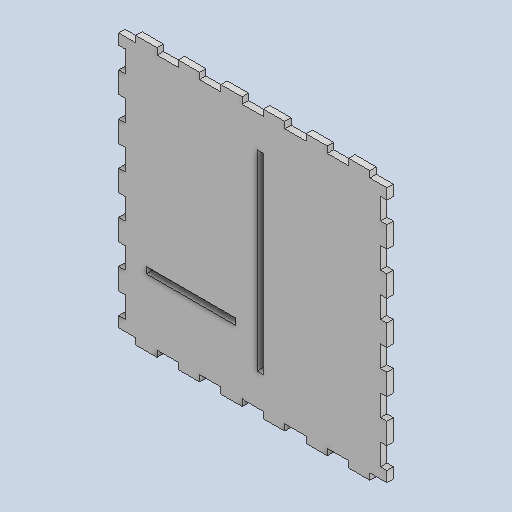
# Autodesk Inventor part: bottom
Saved by Autodesk Inventor 2022 (Build 260153000, 153)
## iProperties
Created: 2022-05-12
Part Number: bottom
Material: Generic
Document SubType Name: Modeling
Designer: Jeanette Guo
Density: 1 g/cm^3
Appearance: Default
Author: Jeanette Guo
Autodesk Inventor part; units mm, degrees
ref_plane "YZ Plane" through (0, 0, 0) normal (1, 0, 0) x (0, 1, 0)
ref_plane "XZ Plane" through (0, 0, 0) normal (0, 1, 0) x (-1, 0, 0)
ref_plane "XY Plane" through (0, 0, 0) normal (0, 0, 1) x (1, 0, 0)
sketch "Sketch2" plane through (0, 0, 0) normal (0, 0, 1) x (1, 0, 0)
  line L0 (109.6174, -113.2467) -> (109.6174, -116.2467) projected
  line L1 (106.6174, -113.2467) -> (106.6174, -116.2467) projected
  line L2 (101.6174, -113.2467) -> (109.6174, -113.2467) projected
  line L3 (101.6174, -116.2467) -> (109.6174, -116.2467) projected
  line L4 (101.6174, -113.2467) -> (101.6174, -116.2467) projected
  line L5 (106.6174, -113.2471) -> (106.6174, -108.2467) projected
  line L6 (109.6174, -113.2471) -> (109.6174, -108.2467) projected
  line L7 (106.6174, -108.2467) -> (106.6174, -98.2467) projected
  line L8 (109.6174, -108.2467) -> (109.6174, -98.2467) projected
  line L9 (109.6174, -98.2467) -> (109.6174, -88.2467) projected
  line L10 (106.6174, -98.2467) -> (106.6174, -88.2467) projected
  line L11 (106.6174, -88.2467) -> (106.6174, -78.2467) projected
  line L12 (109.6174, -88.2467) -> (109.6174, -78.2467) projected
  line L13 (109.6174, -78.2467) -> (109.6174, -68.2467) projected
  line L14 (106.6174, -78.2467) -> (106.6174, -68.2467) projected
  line L15 (106.6174, -78.2467) -> (109.6174, -78.2467) projected
  line L16 (106.6174, -88.2467) -> (109.6174, -88.2467) projected
  line L17 (106.6174, -98.2467) -> (109.6174, -98.2467) projected
  line L18 (106.6174, -108.2467) -> (109.6174, -108.2467) projected
  line L19 (91.6174, -113.2467) -> (91.6174, -116.2467) projected
  line L20 (81.6174, -113.2467) -> (81.6174, -116.2467) projected
  line L21 (71.6174, -113.2467) -> (71.6174, -116.2467) projected
  line L22 (61.6174, -113.2467) -> (61.6174, -116.2467) projected
  line L23 (51.6174, -113.2467) -> (51.6174, -116.2467) projected
  line L24 (106.6174, -68.2467) -> (109.6174, -68.2467)
  line L25 (109.6174, -108.2467) -> (106.6174, -108.2467)
  line L26 (109.6174, -98.2467) -> (106.6174, -98.2467)
  line L27 (109.6174, -88.2467) -> (106.6174, -88.2467)
  line L28 (109.6174, -78.2467) -> (106.6174, -78.2467)
  line L29 (101.6174, -113.2467) -> (101.6174, -116.2467)
  line L30 (91.6174, -113.2467) -> (91.6174, -116.2467)
  line L31 (81.6174, -113.2467) -> (81.6174, -116.2467)
  line L32 (71.6174, -113.2467) -> (71.6174, -116.2467)
  line L33 (61.6174, -113.2467) -> (61.6174, -116.2467)
  line L34 (51.6174, -113.2467) -> (51.6174, -116.2467)
  line L35 (106.6174, -113.2471) -> (106.6174, -113.2467)
  line L36 (106.6174, -113.2467) -> (106.6174, -113.2471)
  line L37 (109.6174, -108.2467) -> (109.6174, -113.2467)
  line L38 (106.6174, -98.2467) -> (106.6174, -108.2467)
  line L39 (106.6174, -108.2467) -> (106.6174, -98.2467)
  line L40 (106.6174, -88.2467) -> (106.6174, -78.2467)
  line L41 (109.6174, -68.2467) -> (109.6174, -78.2467)
  line L42 (109.6174, -88.2467) -> (109.6174, -98.2467)
  line L43 (106.6174, -78.2467) -> (106.6174, -88.2467)
  line L44 (101.6174, -113.2471) -> (106.6174, -113.2471)
  line L45 (101.6174, -116.2467) -> (91.6174, -116.2467)
  line L46 (61.6174, -113.2467) -> (71.6174, -113.2468)
  line L47 (81.6174, -113.2469) -> (91.6174, -113.247)
  line L48 (81.6174, -116.2467) -> (71.6174, -116.2467)
  line L49 (61.6174, -116.2467) -> (51.6174, -116.2467)
  line L50 (106.6174, -53.2467) -> (82.6898, -53.2467) construction
  line L51 (46.6174, -113.2467) -> (46.6174, -98.2467) construction
  line L52 (-8.3826, -113.2467) -> (-8.3826, -116.2467)
  line L53 (1.6174, -113.2467) -> (1.6174, -116.2467)
  line L54 (11.6174, -113.2467) -> (11.6174, -116.2467)
  line L55 (21.6174, -113.2467) -> (21.6174, -116.2467)
  line L56 (31.6174, -113.2467) -> (31.6174, -116.2467)
  line L57 (41.6174, -113.2467) -> (41.6174, -116.2467)
  line L58 (-8.3826, -113.2467) -> (-8.3826, -116.2467)
  line L59 (1.6174, -113.2467) -> (1.6174, -116.2467)
  line L60 (11.6174, -113.2467) -> (11.6174, -116.2467)
  line L61 (21.6174, -113.2467) -> (21.6174, -116.2467)
  line L62 (31.6174, -113.2467) -> (31.6174, -116.2467)
  line L63 (41.6174, -113.2467) -> (41.6174, -116.2467)
  line L64 (-8.3826, -116.2467) -> (1.6174, -116.2467)
  line L65 (11.6174, -116.2467) -> (21.6174, -116.2467)
  line L66 (31.6174, -116.2467) -> (41.6174, -116.2467)
  line L67 (-16.3826, -113.2471) -> (-16.3826, -108.2467)
  line L68 (-16.3826, -98.2467) -> (-16.3826, -88.2467)
  line L69 (-16.3826, -78.2467) -> (-16.3826, -68.2467)
  line L70 (-16.3826, -108.2467) -> (-16.3826, -113.2467)
  line L71 (-16.3826, -68.2467) -> (-16.3826, -78.2467)
  line L72 (-16.3826, -88.2467) -> (-16.3826, -98.2467)
  line L73 (109.6174, 6.7533) -> (109.6174, 6.7538)
  line L74 (106.6174, 6.7533) -> (106.6174, 6.7538)
  line L75 (101.6174, 6.7533) -> (109.6174, 6.7533)
  line L76 (101.6174, 6.7533) -> (101.6174, 9.7533)
  line L77 (106.6174, 6.7538) -> (106.6174, 6.7533)
  line L78 (109.6174, 6.7538) -> (109.6174, 1.7533)
  line L79 (106.6174, 1.7533) -> (106.6174, -8.2467)
  line L80 (109.6174, -8.2467) -> (109.6174, -18.2467)
  line L81 (106.6174, -18.2467) -> (106.6174, -28.2467)
  line L82 (109.6174, -28.2467) -> (109.6174, -38.2467)
  line L83 (106.6174, -28.2467) -> (109.6174, -28.2467)
  line L84 (106.6174, -18.2467) -> (109.6174, -18.2467)
  line L85 (106.6174, -8.2467) -> (109.6174, -8.2467)
  line L86 (106.6174, 1.7533) -> (109.6174, 1.7533)
  line L87 (91.6174, 6.7533) -> (91.6174, 9.7533)
  line L88 (81.6174, 6.7533) -> (81.6174, 9.7533)
  line L89 (71.6174, 6.7533) -> (71.6174, 9.7533)
  line L90 (61.6174, 6.7533) -> (61.6174, 9.7533)
  line L91 (51.6174, 6.7533) -> (51.6174, 9.7533)
  line L92 (106.6174, -38.2467) -> (109.6174, -38.2467)
  line L93 (109.6174, 1.7533) -> (106.6174, 1.7533)
  line L94 (109.6174, -8.2467) -> (106.6174, -8.2467)
  line L95 (109.6174, -18.2467) -> (106.6174, -18.2467)
  line L96 (109.6174, -28.2467) -> (106.6174, -28.2467)
  line L97 (101.6174, 6.7533) -> (101.6174, 9.7533)
  line L98 (91.6174, 6.7533) -> (91.6174, 9.7533)
  line L99 (81.6174, 6.7533) -> (81.6174, 9.7533)
  line L100 (71.6174, 6.7533) -> (71.6174, 9.7533)
  line L101 (61.6174, 6.7533) -> (61.6174, 9.7533)
  line L102 (51.6174, 6.7533) -> (51.6174, 9.7533)
  line L103 (106.6174, 6.7538) -> (106.6174, 6.7533)
  line L104 (106.6174, 6.7533) -> (106.6174, 6.7538)
  line L105 (109.6174, 1.7533) -> (109.6174, 6.7533)
  line L106 (106.6174, -8.2467) -> (106.6174, 1.7533)
  line L107 (106.6174, 1.7533) -> (106.6174, -8.2467)
  line L108 (106.6174, -18.2467) -> (106.6174, -28.2467)
  line L109 (109.6174, -38.2467) -> (109.6174, -28.2467)
  line L110 (109.6174, -18.2467) -> (109.6174, -8.2467)
  line L111 (106.6174, -28.2467) -> (106.6174, -18.2467)
  line L112 (101.6174, 6.7538) -> (106.6174, 6.7538)
  line L113 (101.6174, 9.7533) -> (91.6174, 9.7533)
  line L114 (61.6174, 6.7534) -> (71.6174, 6.7535)
  line L115 (81.6174, 6.7536) -> (91.6174, 6.7537)
  line L116 (81.6174, 9.7533) -> (71.6174, 9.7533)
  line L117 (61.6174, 9.7533) -> (51.6174, 9.7533)
  line L118 (46.6174, 6.7533) -> (46.6174, -8.2467) construction
  line L119 (31.6174, 6.7533) -> (31.6174, 9.7533)
  line L120 (41.6174, 6.7533) -> (41.6174, 9.7533)
  line L121 (31.6174, 6.7533) -> (31.6174, 9.7533)
  line L122 (41.6174, 6.7533) -> (41.6174, 9.7533)
  line L123 (31.6174, 9.7533) -> (41.6174, 9.7533)
  line L124 (-8.3826, 6.7533) -> (-8.3826, 9.7533)
  line L125 (1.6174, 6.7533) -> (1.6174, 9.7533)
  line L126 (11.6174, 6.7533) -> (11.6174, 9.7533)
  line L127 (21.6174, 6.7533) -> (21.6174, 9.7533)
  line L128 (-8.3826, 6.7533) -> (-8.3826, 9.7533)
  line L129 (1.6174, 6.7533) -> (1.6174, 9.7533)
  line L130 (-8.3826, 9.7533) -> (1.6174, 9.7533)
  line L131 (11.6174, 6.7533) -> (11.6174, 9.7533)
  line L132 (21.6174, 6.7533) -> (21.6174, 9.7533)
  line L133 (11.6174, 9.7533) -> (21.6174, 9.7533)
  line L134 (-16.3826, -8.2467) -> (-16.3826, -18.2467)
  line L135 (-16.3826, -18.2467) -> (-16.3826, -8.2467)
  line L136 (-16.3826, 1.7533) -> (-16.3826, 6.7533)
  line L137 (-16.3826, 6.7538) -> (-16.3826, 1.7533)
  line L138 (-16.3826, -28.2467) -> (-16.3826, -38.2467)
  line L139 (-16.3826, -38.2467) -> (-16.3826, -28.2467)
  line L140 (109.6174, -58.2467) -> (106.6174, -58.2467)
  line L141 (109.6174, -58.2467) -> (109.6174, -48.2467)
  line L142 (109.6174, -48.2467) -> (106.6174, -48.2467)
  line L143 (-16.3826, -68.2467) -> (-13.3826, -68.2467)
  line L144 (-16.3826, -58.2467) -> (-13.3826, -58.2467)
  line L145 (-16.3826, -58.2467) -> (-16.3826, -48.2467)
  line L146 (-16.3826, -48.2467) -> (-13.3826, -48.2467)
  line L147 (-16.3826, -38.2467) -> (-13.3826, -38.2467)
  line L148 (-16.3826, -108.2467) -> (-13.3826, -108.2467)
  line L149 (-16.3826, -98.2467) -> (-13.3826, -98.2467)
  line L150 (-16.3826, -88.2467) -> (-13.3826, -88.2467)
  line L151 (-16.3826, -78.2467) -> (-13.3826, -78.2467)
  line L152 (-16.3826, -28.2467) -> (-13.3826, -28.2467)
  line L153 (-16.3826, -18.2467) -> (-13.3826, -18.2467)
  line L154 (-16.3826, -8.2467) -> (-13.3826, -8.2467)
  line L155 (106.6174, -113.2467) -> (106.6174, -113.2471)
  line L156 (106.6174, -113.2471) -> (106.6174, -113.2467)
  line L157 (109.6174, -113.2467) -> (101.6174, -113.2467)
  line L158 (91.6174, -113.2467) -> (81.6174, -113.2467)
  line L159 (71.6174, -113.2467) -> (61.6174, -113.2467)
  line L160 (51.6174, -113.2467) -> (46.6174, -113.2467)
  line L161 (41.6174, -113.2467) -> (46.6174, -113.2467)
  line L162 (21.6174, -113.2467) -> (31.6174, -113.2467)
  line L163 (-16.3826, -113.2467) -> (-8.3826, -113.2467)
  line L164 (1.6174, -113.2467) -> (11.6174, -113.2467)
  line L165 (-13.3826, -98.2467) -> (-13.3826, -108.2467)
  line L166 (-13.3826, -108.2467) -> (-13.3826, -98.2467)
  line L167 (-13.3826, -88.2467) -> (-13.3826, -78.2467)
  line L168 (-13.3826, -78.2467) -> (-13.3826, -88.2467)
  line L169 (-13.3826, -58.2467) -> (-13.3826, -68.2467)
  line L170 (-13.3826, -68.2467) -> (-13.3826, -58.2467)
  line L171 (-13.3826, -48.2467) -> (-13.3826, -38.2467)
  line L172 (-13.3826, -38.2467) -> (-13.3826, -48.2467)
  line L173 (-13.3826, -18.2467) -> (-13.3826, -28.2467)
  line L174 (-13.3826, -28.2467) -> (-13.3826, -18.2467)
  line L175 (-16.3826, 1.7533) -> (-13.3826, 1.7533)
  line L176 (-13.3826, -8.2467) -> (-13.3826, 1.7533)
  line L177 (-13.3826, 1.7533) -> (-13.3826, -8.2467)
  line L178 (-16.3826, 6.7533) -> (-8.3826, 6.7533)
  line L179 (1.6174, 6.7533) -> (11.6174, 6.7533)
  line L180 (21.6174, 6.7533) -> (31.6174, 6.7533)
  line L181 (41.6174, 6.7533) -> (46.6174, 6.7533)
  line L182 (51.6174, 6.7533) -> (46.6174, 6.7533)
  line L183 (71.6174, 6.7533) -> (61.6174, 6.7533)
  line L184 (109.6174, 6.7533) -> (101.6174, 6.7533)
  line L185 (91.6174, 6.7533) -> (81.6174, 6.7533)
  line L186 (106.6174, 6.7533) -> (106.6174, 6.7538)
  line L187 (106.6174, 6.7538) -> (106.6174, 6.7533)
  line L188 (106.6174, 1.7533) -> (106.6174, -8.2467)
  line L189 (106.6174, -8.2467) -> (106.6174, 1.7533)
  line L190 (106.6174, -28.2467) -> (106.6174, -18.2467)
  line L191 (106.6174, -18.2467) -> (106.6174, -28.2467)
  line L192 (106.6174, -38.2467) -> (106.6174, -48.2467)
  line L193 (106.6174, -48.2467) -> (106.6174, -38.2467)
  line L194 (106.6174, -68.2467) -> (106.6174, -58.2467)
  line L195 (106.6174, -58.2467) -> (106.6174, -68.2467)
  line L196 (106.6174, -78.2467) -> (106.6174, -88.2467)
  line L197 (106.6174, -98.2467) -> (106.6174, -108.2467)
  line L198 (106.6174, -108.2467) -> (106.6174, -98.2467)
  line L199 (106.6174, -88.2467) -> (106.6174, -78.2467)
  point P0 (0, 0)
  point P1 (106.6174, -116.2467)
  point P2 (-13.3826, -113.2467)
  constraints: 352 end point, 84 symmetric about line, 44 perpendicular, 32 point on line, 18 collinear, 8 parallel, 5 horizontal, 4 vertical
extrude "Extrusion2" add sketch "Sketch2" along normal blind 3 contours L2 L5 L18 L6 | L2 L4 L45 L19 L47 L20 L48 L21 L46 L22 L49 L23 L160 L161 L57 L66 L56 L162 L55 L65 L54 L164 L53 L64 L52 L163 L67 L148 L165 L149 L68 L150 L167 L151 L69 L143 L169 L144 L145 L146 L171 L147 L138 L152 L173 L153 L134 L154 L176 L175 L136 L178 L124 L130 L125 L179 L126 L133 L127 L180 L119 L123 L120 L181 L182 L91 L117 L90 L114 L89 L116 L88 L115 L87 L113 L76 L75 L78 L86 L79 L85 L80 L84 L81 L83 L82 L92 L192 L142 L141 L140 L194 L14 L11 L10 L7 L5 | L17 L10 L16 L9 | L15 L14 L24 L13
sketch "Sketch3" plane through (0, 0, 3) normal (0, 0, 1) x (1, 0, 0)
  line L0 (51.6174, 4.7533) -> (51.6174, -111.2467) projected
  line L1 (51.6174, 4.7533) -> (48.6174, 4.7533)
  line L2 (41.6174, -113.2467) -> (51.6174, -113.2467) projected
  line L3 (51.6174, -113.2467) -> (51.6174, -53.2467)
  line L4 (51.6174, -53.2467) -> (48.6174, -53.2467)
  line L5 (48.6174, -53.2467) -> (48.6174, -8.2467)
  line L6 (48.6174, -8.2467) -> (51.6174, -8.2467)
  line L7 (48.6174, -53.2467) -> (48.6174, -98.2467)
  line L8 (48.6174, -98.2467) -> (51.6174, -98.2467)
  line L9 (51.6174, -98.2467) -> (51.6174, -8.2467)
  point P0 (0, 0)
  dimension "d20" = 60
  dimension "d21" = 45
  dimension "d22" = 45
  constraints: 16 end point, 4 perpendicular, 3 point on line, 1 collinear, 1 horizontal, 1 midpoint
  measures "d20" distance of L2.end L3.end
  measures "d21" distance of L4.end L5.end
  measures "d22" distance of L4.end L7.end
extrude "Extrusion3" cut sketch "Sketch3" against normal blind 3
sketch "Sketch4" plane through (0, 0, 0) normal (0, 0, -1) x (-1, 0, 0)
  line L0 (-21.6174, -113.2467) -> (-31.6174, -113.2467) projected
  line L1 (13.3826, -58.2467) -> (13.3826, -68.2467) projected
  line L2 (-38.6174, -81.7467) -> (-38.6174, -84.7467)
  line L3 (-48.6174, -98.2467) -> (-48.6174, -8.2467) projected
  line L4 (-38.6174, -84.7467) -> (3.3826, -84.7467)
  circle A0 centre (-68.8966, -83.2467) radius 3 projected
  line L5 (-38.6174, -81.7467) -> (3.3826, -81.7467)
  line L6 (3.3826, -81.7467) -> (3.3826, -84.7467)
  line L7 (13.3826, -78.2467) -> (13.3826, -88.2467) projected
  point P0 (0, 0)
  point P1 (-38.6174, -83.2467)
  dimension "d27" = 3
  dimension "d32" = 42
  dimension "d33" = 42
  dimension "d34" = 10
  dimension "d35" = 10
  constraints: 8 end point, 2 perpendicular, 1 horizontal, 1 horizontal alignment, 1 midpoint, 1 parallel
  measures "d27" distance of L2.start L2.end
  measures "d32" distance of L2.end L4.end
  measures "d33" distance of L2.start L5.end
  measures "d34" distance between parallel lines of L7 L6
  measures "d35" distance between parallel lines of L3 L2
extrude "Extrusion4" cut sketch "Sketch4" against normal blind 10 contours L5 L6 L4 L2
body "Solid2"
